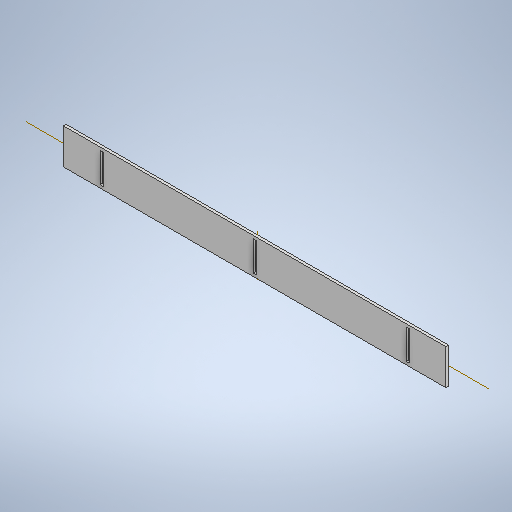
# Autodesk Inventor part: side_wall
Saved by Autodesk Inventor 2025 (Build 290162000, 162)
## iProperties
Created: 2024-04-06
Part Number: side_wall
Material: 일반
Document SubType Name: Modeling
Designer: gmsee
Density: 1 g/cm^3
Appearance: 기본값
Author: gmsee
Autodesk Inventor part; units mm, degrees
ref_plane "YZ Plane" through (0, 0, 0) normal (1, 0, 0) x (0, 1, 0)
ref_plane "XZ Plane" through (0, 0, 0) normal (0, 1, 0) x (-1, 0, 0)
ref_plane "XY Plane" through (0, 0, 0) normal (0, 0, 1) x (1, 0, 0)
sketch "스케치1" plane through (0, 0, 0) normal (0, 0, 1) x (1, 0, 0)
  line L0 (0, 23.25) -> (250, 23.25)
  line L1 (250, 23.25) -> (250, 0)
  line L2 (0, -42.1597) -> (0, 34.1516) projected
  line L3 (-350, 0) -> (350, 0) projected
  line L4 (0, 19.35) -> (1.85, 19.35)
  line L5 (1.85, 19.35) -> (1.85, 0)
  line L6 (198.15, 0) -> (198.15, 19.35)
  line L7 (198.15, 19.35) -> (201.85, 19.35)
  line L8 (201.85, 19.35) -> (201.85, 0)
  line L9 (0, 23.25) -> (-250, 23.25)
  line L10 (-250, 23.25) -> (-250, 0)
  line L11 (0, 19.35) -> (-1.85, 19.35)
  line L12 (-1.85, 19.35) -> (-1.85, 0)
  line L13 (-198.15, 0) -> (-198.15, 19.35)
  line L14 (-198.15, 19.35) -> (-201.85, 19.35)
  line L15 (-201.85, 19.35) -> (-201.85, 0)
  line L16 (0, -23.25) -> (250, -23.25)
  line L17 (250, -23.25) -> (250, 0)
  line L18 (0, 5.2097) -> (0, -31.2581)
  line L19 (0, -19.35) -> (1.85, -19.35)
  line L20 (1.85, -19.35) -> (1.85, 0)
  line L21 (198.15, 0) -> (198.15, -19.35)
  line L22 (198.15, -19.35) -> (201.85, -19.35)
  line L23 (201.85, -19.35) -> (201.85, 0)
  line L24 (0, -23.25) -> (-250, -23.25)
  line L25 (-250, -23.25) -> (-250, 0)
  line L26 (0, -19.35) -> (-1.85, -19.35)
  line L27 (-1.85, -19.35) -> (-1.85, 0)
  line L28 (-198.15, 0) -> (-198.15, -19.35)
  line L29 (-198.15, -19.35) -> (-201.85, -19.35)
  line L30 (-201.85, -19.35) -> (-201.85, 0)
  point P0 (0, 0)
  dimension "d0" = 250
  dimension "d1" = 23.25
  dimension "d2" = 1.85
  dimension "d3" = 3.7
  dimension "d4" = 19.35
  dimension "d5" = 19.35
  dimension "d6" = 48.15
  constraints: 58 end point, 8 point on line, 8 symmetric about line, 4 perpendicular, 2 horizontal, 1 vertical
  measures "d0" distance of L0.start L0.end
  measures "d1" distance of L0.end L1.end
  measures "d2" distance of L4.start L4.end
  measures "d3" distance between parallel lines of L8 L6
  measures "d4" distance of L4.end L5.end
  measures "d5" distance of L6.start L6.end
  measures "d6" distance between parallel lines of L1 L8
extrude "돌출1" add sketch "스케치1" along normal blind 3.5 contours L0 L1 L3 L8 L7 L6 L5 L4 L2 | L2 L11 L12 L3 L13 L14 L15 L10 L9 | L17 L16 L2 L19 L20 L3 L21 L22 L23 | L3 L30 L29 L28 L27 L26 L2 L24 L25
